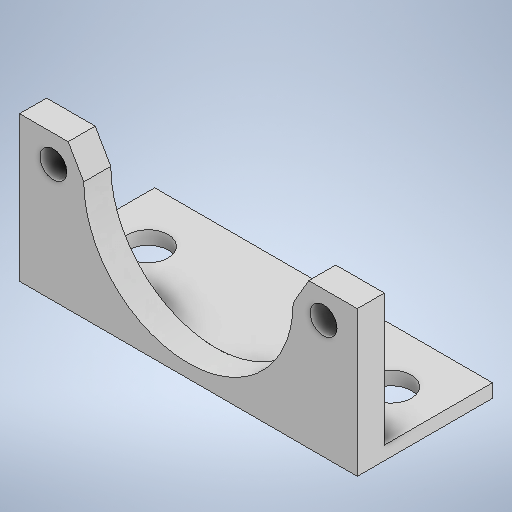
# Autodesk Inventor part: Stepper-D15-S18_Braket
Saved by Autodesk Inventor 2025.3 (Build 293356000, 356)
## iProperties
Created: 2025-06-27
Part Number: Stepper-D15-S18_Braket
Material: 一般
Document SubType Name: Modeling
Designer: yamashita1
Density: 1 g/cm^3
Appearance: 既定
Author: yamashita1
Autodesk Inventor part; units mm, degrees
ref_plane "YZ Plane" through (0, 0, 0) normal (1, 0, 0) x (0, 1, 0)
ref_plane "XZ Plane" through (0, 0, 0) normal (0, 1, 0) x (-1, 0, 0)
ref_plane "XY Plane" through (0, 0, 0) normal (0, 0, 1) x (1, 0, 0)
sketch "スケッチ1" plane through (0, 0, 0) normal (0, 0, 1) x (1, 0, 0)
  line L0 (-12.5, 0) -> (12.5, 0)
  line L1 (12.5, 0) -> (12.5, 10)
  line L2 (12.5, 10) -> (-12.5, 10)
  line L3 (-12.5, 10) -> (-12.5, 0)
  point P0 (0, 0)
  point P1 (0, 0)
  dimension "d0" = 25
  dimension "d1" = 10
  constraints: 8 end point, 2 parallel, 1 coincident, 1 horizontal, 1 midpoint, 1 perpendicular
  measures "d0" distance of L2.end L1.end
  measures "d1" distance of L1.end L0.end
extrude "押し出し1" add sketch "スケッチ1" along normal blind 1
sketch "スケッチ2" plane through (-12.5, 0, 0) normal (0, -1, 0) x (1, 0, 0)
  line L0 (12.5, 0) -> (12.5, 16.3622) construction
  circle A0 centre (12.5, 8.75) radius 7.75
  line L1 (0, 1) -> (25, 1) construction
  line L2 (-3.4099, 8.75) -> (28.4099, 8.75) construction
  circle A1 centre (2.5, 8.75) radius 1
  circle A2 centre (22.5, 8.75) radius 1
  line L3 (0, 1) -> (0, 10.75)
  line L4 (0, 1) -> (25, 1)
  line L5 (25, 1) -> (25, 10.75)
  line L6 (0, 10.75) -> (3.5953, 10.75)
  line L7 (3.5953, 10.75) -> (4.75, 8.75)
  line L8 (25, 10.75) -> (21.4047, 10.75)
  line L9 (21.4047, 10.75) -> (20.25, 8.75)
  point P0 (12.5, 1)
  dimension "d4" = 15.5
  dimension "d5" = 2
  dimension "d6" = 20
  dimension "d8" = 2
  dimension "d9" = 60
  dimension "d10" = 60
  constraints: 18 end point, 6 point on line, 3 centre point, 3 vertical, 2 horizontal, 2 point on circle, 1 collinear, 1 equal radius, 1 midpoint, 1 symmetric about line, 1 tangent
  measures "d4" diameter of A0
  measures "d5" diameter of A1
  measures "d6" distance of A2.centre A1.centre
  measures "d8" distance from line of A2.centre L8
  measures "d9" angle of L2 L9
  measures "d10" angle of L2 L7
extrude "押し出し2" add sketch "スケッチ2" against normal blind 2 contours L9 L8 L5 L4 A0 | A0 L4 L3 L6 L7
sketch "スケッチ4" plane through (0, 0, 0) normal (0, 0, -1) x (-1, 0, 0)
  line L0 (18.7059, 6) -> (-18.7059, 6) construction
  line L1 (0, -10.402) -> (0, 10.402) construction
  line L2 (12.5, 0) -> (-12.5, 0) construction
  point P0 (0, 0)
  point P1 (0, 0)
  point P2 (0, 6)
  point P3 (9, 6)
  point P4 (-9, 6)
  dimension "d17" = 18
  dimension "d18" = 6
  constraints: 4 end point, 3 midpoint, 3 point on line, 1 horizontal, 1 symmetric about line, 1 vertical
  measures "d17" distance of point (-9, 6) point (9, 6)
  measures "d18" distance between parallel lines of L2 L0
hole "穴1" at (-9, 6, 0) at (9, 6, 0) direction (0, 0, 1) diameter 3 end through all
equation "\"d10\" = d9"
